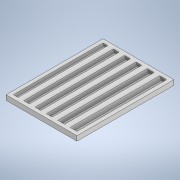
# Autodesk Inventor part: punchTray
Saved by Autodesk Inventor 2020.2 (Build 242310000, 310)
## iProperties
Created: 2019-12-07
Part Number: punchTray
Material: Generic
Document SubType Name: Modeling
Designer: robst
Density: 1 g/cm^3
Appearance: Default
Author: robst
Autodesk Inventor part; units mm, degrees
ref_plane "YZ Plane" through (0, 0, 0) normal (1, 0, 0) x (0, 1, 0)
ref_plane "XZ Plane" through (0, 0, 0) normal (0, 1, 0) x (-1, 0, 0)
ref_plane "XY Plane" through (0, 0, 0) normal (0, 0, 1) x (1, 0, 0)
sketch "Sketch3" plane through (0, 0, 0) normal (0, 0, 1) x (1, 0, 0)
  line L0 (-60.4011, -4.0957) -> (60.4011, -4.0957)
  line L1 (60.4011, -4.0957) -> (60.4011, 4.0957)
  line L2 (60.4011, 4.0957) -> (-60.4011, 4.0957)
  line L3 (-60.4011, 4.0957) -> (-60.4011, -4.0957)
  line L4 (-60.4011, -4.0957) -> (60.4011, 4.0957) construction
  line L5 (60.4011, -4.0957) -> (-60.4011, 4.0957) construction
  line L6 (54.0511, 4.0957) -> (51.1548, -0.9208)
  line L7 (51.1548, -0.9208) -> (45.3623, -0.9208)
  line L8 (45.3623, -0.9208) -> (42.466, 4.0957)
  line L9 (42.466, 4.0957) -> (45.3623, 9.1122)
  line L10 (45.3623, 9.1122) -> (51.1548, 9.1123)
  line L11 (51.1548, 9.1123) -> (54.0511, 4.0957)
  line L12 (32.941, 4.0957) -> (30.0447, -0.9208)
  line L13 (30.0447, -0.9208) -> (24.2522, -0.9208)
  line L14 (24.2522, -0.9208) -> (21.3559, 4.0957)
  line L15 (21.3559, 4.0957) -> (24.2522, 9.1122)
  line L16 (24.2522, 9.1122) -> (30.0447, 9.1122)
  line L17 (30.0447, 9.1122) -> (32.941, 4.0957)
  line L18 (0, 0) -> (0, 4.0957) construction
  line L19 (11.8309, 4.0957) -> (9.3745, -0.1588)
  line L20 (9.3745, -0.1588) -> (4.4619, -0.1588)
  line L21 (4.4619, -0.1588) -> (2.0055, 4.0957)
  line L22 (2.0055, 4.0957) -> (4.4619, 8.3502)
  line L23 (4.4619, 8.3502) -> (9.3745, 8.3502)
  line L24 (9.3745, 8.3502) -> (11.8309, 4.0957)
  line L25 (-7.5195, 4.0957) -> (-9.9758, -0.1588)
  line L26 (-9.9758, -0.1588) -> (-14.8885, -0.1588)
  line L27 (-14.8885, -0.1588) -> (-17.3448, 4.0957)
  line L28 (-17.3448, 4.0957) -> (-14.8885, 8.3502)
  line L29 (-14.8885, 8.3502) -> (-9.9758, 8.3502)
  line L30 (-9.9758, 8.3502) -> (-7.5195, 4.0957)
  line L31 (-26.8698, 4.0957) -> (-29.3041, -0.1207)
  line L32 (-29.3041, -0.1207) -> (-34.1728, -0.1206)
  line L33 (-34.1728, -0.1206) -> (-36.6072, 4.0958)
  line L34 (-36.6072, 4.0958) -> (-34.1728, 8.3121)
  line L35 (-34.1728, 8.3121) -> (-29.3041, 8.3121)
  line L36 (-29.3041, 8.3121) -> (-26.8698, 4.0957)
  line L37 (-46.1322, 4.0957) -> (-48.1119, 0.6667)
  line L38 (-48.1119, 0.6667) -> (-52.0714, 0.6667)
  line L39 (-52.0714, 0.6667) -> (-54.0511, 4.0957)
  line L40 (-54.0511, 4.0957) -> (-52.0714, 7.5247)
  line L41 (-52.0714, 7.5247) -> (-48.1119, 7.5248)
  line L42 (-48.1119, 7.5248) -> (-46.1322, 4.0957)
  point P0 (48.2585, 4.0957)
  point P1 (27.1484, 4.0957)
  point P2 (42.466, 4.0957)
  point P3 (21.3559, 4.0957)
  point P4 (6.9182, 4.0957)
  point P5 (-12.4321, 4.0957)
  point P6 (-31.7385, 4.0957)
  point P7 (-50.0916, 4.0957)
  point P8 (2.0055, 4.0957)
  point P9 (-17.3448, 4.0957)
  point P10 (-36.6072, 4.0957)
  point P11 (-54.0511, 4.0957)
  dimension "d7" = 10.033
  dimension "d8" = 10.033
  dimension "d13" = 6.35
  dimension "d14" = 9.525
  dimension "d15" = 8.509
  dimension "d16" = 9.525
  dimension "d17" = 8.509
  dimension "d18" = 9.525
  dimension "d19" = 8.4328
  dimension "d20" = 9.525
  dimension "d21" = 9.525
  dimension "d22" = 6.858
  dimension "d23" = 6.35
  dimension "d24" = 3.175
  constraints: 84 end point, 2 horizontal, 2 midpoint, 1 parallel, 1 perpendicular, 94 other
  measures "d7" distance between parallel lines of L7 L10
  measures "d8" distance between parallel lines of L13 L16
  measures "d13" distance of L6.start L1.end
  measures "d14" distance of L8.end L12.start
  measures "d15" distance between parallel lines of L20 L23
  measures "d16" distance of L14.end L19.start
  measures "d17" distance between parallel lines of L26 L29
  measures "d18" distance of L21.end L25.start
  measures "d19" distance between parallel lines of L32 L35
  measures "d20" distance of L27.end L31.start
  measures "d21" distance of L33.end L37.start
  measures "d22" distance between parallel lines of L38 L41
  measures "d23" distance from line of L39.end L3
  measures "d24" distance between parallel lines of L0 L7
extrude "Extrusion3" add sketch "Sketch3" against normal blind 152.4 contours L3 L2 L39 L38 L37 L33 L32 L31 L27 L26 L25 L21 L20 L19 L14 L13 L12 L8 L7 L6 L1 L0
sketch "Sketch4" plane through (0, 0, 0) normal (0, 0, 1) x (1, 0, 0)
  line L0 (60.4011, -4.0957) -> (-60.4011, -4.0957) projected
  line L1 (60.4011, 4.0957) -> (60.4011, -4.0957) projected
  line L2 (-60.4011, -4.0957) -> (60.4011, -4.0957)
  line L3 (60.4011, -4.0957) -> (60.4011, 4.0957)
  line L4 (60.4011, 4.0957) -> (-60.4011, 4.0957)
  line L5 (-60.4011, 4.0957) -> (-60.4011, -4.0957)
  point P0 (0, 0)
  constraints: 8 end point, 2 parallel, 1 horizontal, 1 perpendicular
extrude "Extrusion4" add sketch "Sketch4" along normal blind 6.35
sketch "Sketch5" plane through (0, 0, -152.4) normal (0, 0, -1) x (-1, 0, 0)
  line L0 (-60.4011, 4.0957) -> (-60.4011, -4.0957) projected
  line L1 (60.4011, 4.0957) -> (54.0511, 4.0957) projected
  line L2 (-60.4011, -4.0957) -> (60.4011, -4.0957)
  line L3 (60.4011, -4.0957) -> (60.4011, 4.0957)
  line L4 (60.4011, 4.0957) -> (-60.4011, 4.0957)
  line L5 (-60.4011, 4.0957) -> (-60.4011, -4.0957)
  point P0 (0, 0)
  constraints: 8 end point, 2 parallel, 1 horizontal, 1 perpendicular
extrude "Extrusion5" add sketch "Sketch5" along normal blind 6.35
equation "\"d14\" = gapBetweenParts"
equation "\"d16\" = gapBetweenParts"
equation "\"d18\" = gapBetweenParts"
equation "\"d20\" = gapBetweenParts"
equation "\"d21\" = gapBetweenParts"
equation "\"gapBetweenParts\" = 9.525"
body "Solid3"
